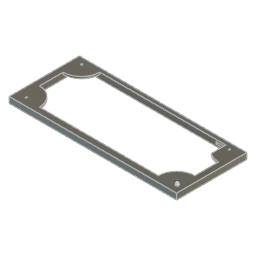
case keyboard mariboard (Autodesk Fusion 360 design; units mm, degrees)
part number: 2026-09-02-15-03-32-432
Autodesk Fusion 360 part; units mm, degrees
sketch "Sketch1" plane through (0, 0, 0) normal (0, 0, 1) x (1, 0, 0)
  line L0 (0, 0) -> (383, 0)
  line L1 (383, 0) -> (383, 148.5)
  line L2 (383, 148.5) -> (0, 148.5)
  line L3 (0, 148.5) -> (0, 0)
  line L4 (-15, 158.5) -> (398, 158.5)
  line L5 (398, 158.5) -> (398, -15)
  line L6 (398, -15) -> (-15, -15)
  line L7 (-15, -15) -> (-15, 158.5)
  circle A0 centre (0, 148.5) radius 45
  circle A1 centre (0, 0) radius 45
  circle A2 centre (383, 0) radius 45
  circle A3 centre (383, 148.5) radius 45
  line L8 (332, 158.5) -> (356, 158.5)
  line L9 (356, 158.5) -> (356, 148.5)
  line L10 (356, 148.5) -> (332, 148.5)
  line L11 (332, 148.5) -> (332, 158.5)
  circle A4 centre (6, 143) radius 3
  circle A5 centre (8.5, 4.25) radius 3
  circle A6 centre (374.8, 6.25) radius 3
  circle A7 centre (370, 143.25) radius 3
  line L12 (356, 148.5) -> (332, 148.5)
  line L13 (332, 148.5) -> (332, 107)
  line L14 (332, 107) -> (356, 107)
  line L15 (356, 107) -> (356, 148.5)
  dimension "d1" = 383
  dimension "d2" = 148.5
  dimension "d3" = 15
  dimension "d4" = 15
  dimension "d5" = 15
  dimension "d6" = 10
  dimension "d7" = 90
  dimension "d8" = 90
  dimension "d9" = 90
  dimension "d10" = 90
  dimension "d11" = 24
  dimension "d12" = 27
  dimension "d13" = 10
  dimension "d14" = 6
  dimension "d15" = 5.5
  dimension "d16" = 6
  dimension "d17" = 6
  dimension "d18" = 8.5
  dimension "d19" = 4.25
  dimension "d20" = 6
  dimension "d21" = 6.25
  dimension "d22" = 8.2
  dimension "d23" = 6
  dimension "d24" = 5.25
  dimension "d25" = 13
  constraint horizontal L0
  constraint vertical L1
  constraint horizontal L2
  constraint vertical L3
  constraint coincident L0.start L3.end
  constraint horizontal L4
  constraint vertical L5
  constraint horizontal L6
  constraint vertical L7
  constraint coincident L2.end L3.start
  constraint coincident L0.end L1.start
  constraint coincident L1.end L2.start
  constraint horizontal L8
  constraint vertical L9
  constraint horizontal L10
  constraint vertical L11
  constraint coincident L4 L8.start
  constraint horizontal L12
  constraint vertical L13
  constraint horizontal L14
  constraint vertical L15
  measures "d1" distance of L0.start L0.end
  measures "d2" distance of L0.start L2.end
  measures "d3" distance of L1 L5
  measures "d4" distance of L3 L7
  measures "d5" distance of L0 L6
  measures "d6" distance of L2 L4
  measures "d7" diameter of A0
  measures "d8" diameter of A1
  measures "d9" diameter of A2
  measures "d10" diameter of A3
  measures "d11" distance of L8.start L8.end
  measures "d12" distance of L1.end L9
  measures "d13" distance of L8.start L10.end
  measures "d14" diameter of A4
  measures "d15" distance of L2 A4.centre
  measures "d16" distance of L3 A4.centre
  measures "d17" diameter of A5
  measures "d18" distance of L3 A5.centre
  measures "d19" distance of L0 A5.centre
  measures "d20" diameter of A6
  measures "d21" distance of L0 A6.centre
  measures "d22" distance of L1 A6.centre
  measures "d23" diameter of A7
  measures "d24" distance of L2 A7.centre
  measures "d25" distance of L1 A7.centre
extrude "Extrude1" add sketch "Sketch1" along normal blind 5 contours L0 L3 A1 | L0 L3 L6 L7 A1 | L0 L6 A1 A2 | L3 L7 A0 A1 | L0 L1 A2 | L0 L1 L5 L6 A2 | L2 L3 L4 L7 A0 | L2 L3 A0 | L1 L5 A2 A3 | L2 L4 A0 L11 | L1 L2 A3 L15 | L1 L2 L4 L5 A3 L9 makes body 1
sketch "Sketch2" plane through (0, 0, 0) normal (0, 0, -1) x (1, 0, 0)
  circle A0 centre (374.8, -6.25) radius 3
  circle A1 centre (8.5, -4.25) radius 3
  circle A2 centre (6, -143) radius 3
  circle A3 centre (370, -143.25) radius 3
  line L0 (356, -112.5) -> (356, -158.5)
  line L1 (356, -158.5) -> (398, -158.5)
  line L2 (398, -158.5) -> (398, 15)
  line L3 (398, 15) -> (-15, 15)
  line L4 (-15, 15) -> (-15, -158.5)
  line L5 (-15, -158.5) -> (332, -158.5)
  line L6 (332, -158.5) -> (332, -148.5)
  line L7 (332, -148.5) -> (45, -148.5)
  arc A4 (45, -148.5) -> (0, -103.5) centre (0, -148.5) ccw
  line L8 (0, -103.5) -> (0, -45)
  arc A5 (0, -45) -> (45, 0) centre (0, 0) ccw
  line L9 (45, 0) -> (338, 0)
  arc A6 (338, 0) -> (383, -45) centre (383, 0) ccw
  line L10 (383, -45) -> (383, -103.5)
  arc A7 (383, -103.5) -> (356, -112.5) centre (383, -148.5) ccw
  line L11 (356, -158.5) -> (332, -158.5)
  line L12 (332, -158.5) -> (332, -148.5)
  line L13 (332, -148.5) -> (356, -148.5)
  line L14 (356, -148.5) -> (356, -158.5)
  constraint horizontal L11
  constraint vertical L12
  constraint horizontal L13
  constraint vertical L14
  constraint coincident L6.end L7.start
  constraint coincident L0.end L1.start
extrude "Extrude2" add sketch "Sketch2" along normal blind 5 separate body contours L0 L6 L11 L12 L13 L14 makes body 2
sketch "Sketch3" plane through (0, 0, 0) normal (0, 0, -1) x (1, 0, 0)
  circle A0 centre (374.8, -6.25) radius 3
  circle A1 centre (8.5, -4.25) radius 3
  circle A2 centre (6, -143) radius 3
  circle A3 centre (370, -143.25) radius 3
  line L0 (356, -112.5) -> (356, -158.5)
  line L1 (356, -158.5) -> (398, -158.5)
  line L2 (398, -158.5) -> (398, 15)
  line L3 (398, 15) -> (-15, 15)
  line L4 (-15, 15) -> (-15, -158.5)
  line L5 (-15, -158.5) -> (332, -158.5)
  line L6 (332, -158.5) -> (332, -148.5)
  line L7 (332, -148.5) -> (45, -148.5)
  arc A4 (45, -148.5) -> (0, -103.5) centre (0, -148.5) ccw
  line L8 (0, -103.5) -> (0, -45)
  arc A5 (0, -45) -> (45, 0) centre (0, 0) ccw
  line L9 (45, 0) -> (338, 0)
  arc A6 (338, 0) -> (383, -45) centre (383, 0) ccw
  line L10 (383, -45) -> (383, -103.5)
  arc A7 (383, -103.5) -> (356, -112.5) centre (383, -148.5) ccw
  line L11 (383, 0) -> (0, 0)
  line L12 (0, 0) -> (0, -148.5)
  line L13 (0, -148.5) -> (383, -148.5)
  line L14 (383, -148.5) -> (383, 0)
  line L15 (-15, -158.5) -> (398, -158.5)
  line L16 (398, -158.5) -> (398, 15)
  line L17 (398, 15) -> (-15, 15)
  line L18 (-15, 15) -> (-15, -158.5)
  constraint horizontal L11
  constraint vertical L12
  constraint horizontal L13
  constraint vertical L14
  constraint coincident A4.centre L12.end
  constraint coincident A6.centre L11.start
  constraint horizontal L15
  constraint vertical L16
  constraint horizontal L17
  constraint vertical L18
  constraint coincident L2.end L3.start
  constraint coincident L4.end L5.start
extrude "Extrude3" add 1 faces at (348, 155.1667, -5) along direction (0, 0, -1) blind 15 on bodies 2 bodies 2
extrude "Extrude4" add sketch "Sketch3" along normal blind 10 contours L0 L1 L2 L3 L4 L5 L6 L7 L8 L9 L10 L11 L12 L13 L14 L15 L16 L17 L18 bodies 1 2
sketch "Sketch4" plane through (0, 0, -20) normal (0, 0, -1) x (1, 0, 0)
  line L0 (356, -148.5) -> (332, -148.5)
  line L1 (332, -148.5) -> (332, -158.5)
  line L2 (332, -158.5) -> (356, -158.5)
  line L3 (356, -158.5) -> (356, -148.5)
sketch "Sketch5" plane through (0, 0, -20) normal (0, 0, -1) x (1, 0, 0)
extrude "Extrude5" cut sketch "Sketch4" against normal blind 10 bodies 1
extrude "Extrude6" add 1 faces at (340, 151.8333, 0) along direction (0, 0, 1) blind 5 on bodies 1 bodies 1
sketch "Sketch6" plane through (0, 158.5, 0) normal (0, 1, 0) x (-1, 0, 0)
  line L0 (-398, -10) -> (15, -10)
  line L1 (15, -10) -> (15, 5)
  line L2 (15, 5) -> (-398, 5)
  line L3 (-398, 5) -> (-398, -10)
sketch "Sketch7" plane through (0, 158.5, 0) normal (0, 1, 0) x (-1, 0, 0)
  line L0 (-356, 0) -> (-332, 0)
  line L1 (-332, 0) -> (-332, -5)
  line L2 (-332, -5) -> (-356, -5)
  line L3 (-356, -5) -> (-356, 0)
  line L4 (-398, 5) -> (-398, -10)
  line L5 (15, 5) -> (-398, 5)
  line L6 (-398, -10) -> (15, -10)
  dimension "d38" = 24
  dimension "d39" = 5
  dimension "d40" = 42
  dimension "d41" = 5
  dimension "d42" = 5
  constraint horizontal L0
  constraint vertical L1
  constraint horizontal L2
  constraint vertical L3
  measures "d38" distance of L0.start L0.end
  measures "d39" distance of L0.start L2.end
  measures "d40" distance of L3 L4
  measures "d41" distance of L0 L5
  measures "d42" distance of L2 L6
extrude "Extrude7" cut sketch "Sketch7" against normal blind 15 bodies 1
sketch "Sketch8" plane through (0, -15, 0) normal (0, -1, 0) x (1, 0, 0)
  line L0 (398, -10) -> (398, 5)
  line L1 (398, 5) -> (-15, 5)
  line L2 (-15, 5) -> (-15, -10)
  line L3 (-15, -10) -> (398, -10)
sketch "Sketch9" plane through (0, 0, 5) normal (0, 0, 1) x (-1, 0, 0)
  line L0 (-356, -148.5) -> (-356, -112.5)
  arc A0 (-356, -112.5) -> (-383, -103.5) centre (-383, -148.5) ccw
  line L1 (-383, -103.5) -> (-383, -45)
  arc A1 (-383, -45) -> (-338, 0) centre (-383, 0) ccw
  line L2 (-338, 0) -> (-45, 0)
  arc A2 (-45, 0) -> (0, -45) centre (0, 0) ccw
  line L3 (0, -45) -> (0, -103.5)
  arc A3 (0, -103.5) -> (-45, -148.5) centre (0, -148.5) ccw
  line L4 (-45, -148.5) -> (-356, -148.5)
  circle A4 centre (-374.8, -6.25) radius 3
  circle A5 centre (-8.5, -4.25) radius 3
  circle A6 centre (-6, -143) radius 3
  circle A7 centre (-370, -143.25) radius 3
  line L5 (-398, -158.5) -> (15, -158.5)
  line L6 (15, -158.5) -> (15, 15)
  line L7 (15, 15) -> (-398, 15)
  line L8 (-398, 15) -> (-398, -158.5)
  circle A8 centre (-8.5, -4.25) radius 2
  circle A9 centre (-6, -143) radius 2
  circle A10 centre (-370, -143.25) radius 2
  circle A11 centre (-374.8, -6.25) radius 2
  dimension "d45" = 4
  dimension "d46" = 4
  dimension "d47" = 4
  dimension "d48" = 4
  constraint concentric A5 A8
  constraint concentric A6 A9
  constraint concentric A7 A10
  constraint concentric A4 A11
  measures "d45" diameter of A8
  measures "d46" diameter of A9
  measures "d47" diameter of A10
  measures "d48" diameter of A11
delete_face "DeleteFace1" 1 faces at (370.8125, 146.1379, 3.3333) on bodies 1
delete_face "DeleteFace2" 1 faces at (8.8191, 144.0261, 3.3333) on bodies 1
delete_face "DeleteFace3" 1 faces at (11.4963, 4.1005, 3.3333) on bodies 1
extrude "Extrude8" cut sketch "Sketch9" against normal blind 15 contours A8 | A9 | A10 | A11 bodies 1
sketch "Sketch10" plane through (0, 0, 5) normal (0, 0, 1) x (-1, 0, 0)
  circle A0 centre (-6, -143) radius 2
  circle A1 centre (-8.5, -4.25) radius 2
  circle A2 centre (-370, -143.25) radius 2
  line L0 (-356, -148.5) -> (-356, -112.5)
  arc A3 (-356, -112.5) -> (-383, -103.5) centre (-383, -148.5) ccw
  line L1 (-383, -103.5) -> (-383, -45)
  arc A4 (-383, -45) -> (-338, 0) centre (-383, 0) ccw
  line L2 (-338, 0) -> (-45, 0)
  arc A5 (-45, 0) -> (0, -45) centre (0, 0) ccw
  line L3 (0, -45) -> (0, -103.5)
  arc A6 (0, -103.5) -> (-45, -148.5) centre (0, -148.5) ccw
  line L4 (-45, -148.5) -> (-356, -148.5)
  circle A7 centre (-374.8, -6.25) radius 3
  line L5 (-398, -158.5) -> (15, -158.5)
  line L6 (15, -158.5) -> (15, 15)
  line L7 (15, 15) -> (-398, 15)
  line L8 (-398, 15) -> (-398, -158.5)
  circle A8 centre (-374.8, -6.25) radius 2
  dimension "d51" = 4
  constraint concentric A7 A8
  measures "d51" diameter of A8
delete_face "DeleteFace4" 1 faces at (376.1686, 8.9196, 3.3333) on bodies 1
extrude "Extrude9" add sketch "Sketch10" against normal blind 15 contours A2 bodies 1
extrude "Extrude10" cut 1 faces at (370.4157, 143.9699, -10) along direction (0, 0, 1) blind 15 on bodies 1 bodies 1
sketch "Sketch11" plane through (0, 0, 0) normal (0, 0, -1) x (1, 0, 0)
  line L0 (383, 0) -> (338, 0)
  arc A0 (338, 0) -> (383, -45) centre (383, 0) ccw
  line L1 (383, -45) -> (383, 0)
  circle A1 centre (374.8, -10) radius 2
  dimension "d56" = 4
  dimension "d57" = 8.2
  dimension "d58" = 10
  measures "d56" diameter of A1
  measures "d57" distance of L1 A1.centre
  measures "d58" distance of L0 A1.centre
sketch "Sketch12" plane through (0, 0, 5) normal (0, 0, 1) x (-1, 0, 0)
  circle A0 centre (-370, -143.25) radius 2
  circle A1 centre (-6, -143) radius 2
  circle A2 centre (-8.5, -4.25) radius 2
  line L0 (-356, -148.5) -> (-356, -112.5)
  arc A3 (-356, -112.5) -> (-383, -103.5) centre (-383, -148.5) ccw
  line L1 (-383, -103.5) -> (-383, -45)
  arc A4 (-383, -45) -> (-338, 0) centre (-383, 0) ccw
  line L2 (-338, 0) -> (-45, 0)
  arc A5 (-45, 0) -> (0, -45) centre (0, 0) ccw
  line L3 (0, -45) -> (0, -103.5)
  arc A6 (0, -103.5) -> (-45, -148.5) centre (0, -148.5) ccw
  line L4 (-45, -148.5) -> (-356, -148.5)
  line L5 (-398, -158.5) -> (15, -158.5)
  line L6 (15, -158.5) -> (15, 15)
  line L7 (15, 15) -> (-398, 15)
  line L8 (-398, 15) -> (-398, -158.5)
  circle A7 centre (-374.8, -10) radius 2
  dimension "d59" = 4
  measures "d59" diameter of A7
extrude "Extrude11" cut sketch "Sketch12" against normal blind 1 contours A0 | A1 | A2 | A7 bodies 1
extrude "Extrude12" cut 1 faces at (374.1408, 10.0994, 4) along direction (0, 0, -1) blind 7 on bodies 1 bodies 1
